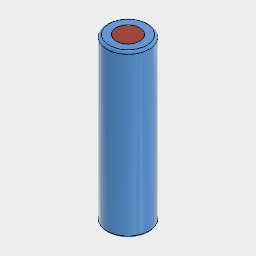
1781 2200mAh Battery (Autodesk Fusion 360 design; units mm, degrees)
Autodesk Fusion 360 part; units mm, degrees
sketch "Sketch1" plane through (0, 0, 0) normal (0, 0, 1) x (1, 0, 0)
  circle A0 centre (0, 0) radius 9
  circle A1 centre (0, 0) radius 5
  dimension "d1" = 18
  dimension "d5" = 10
  measures "d1" diameter of A0
  measures "d5" diameter of A1
extrude "Extrude1" add sketch "Sketch1" along normal blind 69 contours A0 | A1 makes body 1
fillet "Fillet1" radius 1 2 edges at (-8.3909, -3.2545, 69) (-8.3909, -3.2545, 0) on bodies 1
extrude "Extrude2" cut sketch "Sketch1" along normal up to surface (69 mm away) contours A1 bodies 1
extrude "Extrude3" add sketch "Sketch1" along normal up to surface (69 mm away) separate body contours A1 makes body 2
